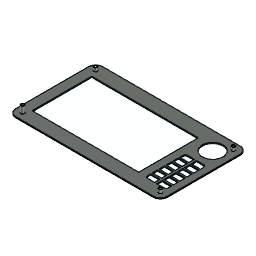
Nexus desk front (Autodesk Fusion 360 design; units mm, degrees)
part number: 2026-05-24-07-28-20-931
Autodesk Fusion 360 part; units mm, degrees
sketch "Sketch1" plane through (0, 0, 0) normal (0, 0, 1) x (1, 0, 0)
  line L0 (20, 40) -> (220, 40)
  line L1 (230, 30) -> (230, -76)
  line L2 (220, -86) -> (20, -86)
  line L3 (10, -76) -> (10, 30)
  arc A0 (20, 40) -> (10, 30) centre (20, 30) ccw
  arc A1 (230, 30) -> (220, 40) centre (220, 30) ccw
  arc A2 (10, -76) -> (20, -86) centre (20, -76) ccw
  arc A3 (220, -86) -> (230, -76) centre (220, -76) ccw
  line L4 (24.5203, 19.9433) -> (179.0203, 19.9433)
  line L5 (179.0203, 19.9433) -> (179.0203, -66.4567)
  line L6 (24.5203, 19.9433) -> (24.5203, -66.4567)
  line L7 (24.5203, -66.4567) -> (179.0203, -66.4567)
  circle A4 centre (205.8832, 13.8979) radius 15
  arc A5 (193, -10) -> (190, -13) centre (193, -13) ccw
  arc A6 (220, -13) -> (217, -10) centre (217, -13) ccw
  arc A7 (190, -64.7013) -> (193, -67.7013) centre (193, -64.7013) ccw
  arc A8 (217, -67.7013) -> (220, -64.7013) centre (217, -64.7013) ccw
  line L8 (203.1137, -60) -> (203.1137, -67.7013)
  line L9 (206.5757, -60) -> (206.5757, -67.7013)
  line L10 (190, -47.6988) -> (203.1137, -47.6988)
  line L11 (206.5757, -47.6988) -> (220, -47.6988)
  line L12 (190, -50) -> (203.1137, -50)
  line L13 (206.5757, -50) -> (220, -50)
  line L14 (203.1137, -50) -> (203.1137, -57.3154)
  line L15 (206.5757, -50) -> (206.5757, -57.3154)
  line L16 (190, -57.3154) -> (203.1137, -57.3154)
  line L17 (206.5757, -57.3154) -> (220, -57.3154)
  line L18 (190, -60) -> (203.1137, -60)
  line L19 (206.5757, -60) -> (220, -60)
  line L20 (190, -64.7013) -> (190, -60)
  line L21 (190, -57.3154) -> (190, -50)
  line L22 (190, -47.6988) -> (190, -40)
  line L23 (203.1137, -40) -> (203.1137, -47.6988)
  line L24 (190, -37.5051) -> (203.1137, -37.5051)
  line L25 (206.5757, -37.5051) -> (220, -37.5051)
  line L26 (190, -40) -> (203.1137, -40)
  line L27 (206.5757, -40) -> (220, -40)
  line L28 (206.5757, -40) -> (206.5757, -47.6988)
  line L29 (220, -50) -> (220, -57.3154)
  line L30 (220, -60) -> (220, -64.7013)
  line L31 (220, -40) -> (220, -47.6988)
  line L32 (193, -67.7013) -> (203.1137, -67.7013)
  line L33 (206.5757, -67.7013) -> (217, -67.7013)
  line L34 (203.1137, -30) -> (203.1137, -37.5051)
  line L35 (190, -27.6962) -> (203.1137, -27.6962)
  line L36 (206.5757, -27.6962) -> (220, -27.6962)
  line L37 (190, -30) -> (203.1137, -30)
  line L38 (206.5757, -30) -> (220, -30)
  line L39 (206.5757, -30) -> (206.5757, -37.5051)
  line L40 (220, -30) -> (220, -37.5051)
  line L41 (190, -37.5051) -> (190, -30)
  line L42 (190, -27.6962) -> (190, -20)
  line L43 (190, -17.8872) -> (190, -13)
  line L44 (203.1137, -10) -> (203.1137, -17.8872)
  line L45 (203.1137, -20) -> (203.1137, -27.6962)
  line L46 (190, -17.8872) -> (203.1137, -17.8872)
  line L47 (206.5757, -17.8872) -> (220, -17.8872)
  line L48 (190, -20) -> (203.1137, -20)
  line L49 (206.5757, -20) -> (220, -20)
  line L50 (206.5757, -10) -> (206.5757, -17.8872)
  line L51 (206.5757, -20) -> (206.5757, -27.6962)
  line L52 (220, -13) -> (220, -17.8872)
  line L53 (220, -20) -> (220, -27.6962)
  line L54 (193, -10) -> (203.1137, -10)
  line L55 (206.5757, -10) -> (217, -10)
  point P0 (10, 40)
  point P1 (230, 40)
  point P2 (10, -86)
  dimension "d1" = 220
  dimension "d2" = 126
  dimension "d3" = 10
  dimension "d4" = 10
  dimension "d5" = 10
  dimension "d6" = 154.5
  dimension "d7" = 86.4
  dimension "d8" = 86.4
  dimension "d9" = 30
  dimension "d10" = 3
  constraint horizontal L0
  constraint vertical L1
  constraint horizontal L2
  constraint vertical L3
  constraint coincident P0 L0
  constraint coincident P0 L3
  constraint tangent L0 A0
  constraint tangent L3 A0
  constraint coincident P1 L0
  constraint coincident P1 L1
  constraint tangent L0 A1
  constraint tangent L1 A1
  constraint coincident P2 L2
  constraint coincident P2 L3
  constraint tangent L2 A2
  constraint tangent L3 A2
  constraint tangent L1 A3
  constraint tangent L2 A3
  constraint equal A2 A3
  constraint perpendicular L3 L4
  constraint perpendicular L4 L5
  constraint perpendicular L4 L6
  constraint horizontal L54
  constraint vertical L52
  constraint vertical L20
  constraint perpendicular L47 L52
  constraint perpendicular L49 L53
  constraint perpendicular L36 L53
  constraint perpendicular L38 L40
  constraint perpendicular L25 L40
  constraint perpendicular L11 L31
  constraint perpendicular L13 L29
  constraint perpendicular L17 L29
  constraint perpendicular L19 L30
  constraint perpendicular L30 L33
  constraint perpendicular L8 L32
  constraint perpendicular L9 L19
  constraint tangent A5 L54
  constraint tangent A5 L43
  constraint tangent A6 L55
  constraint tangent A6 L52
  constraint equal A5 A6
  constraint tangent A7 L20
  constraint tangent A7 L32
  constraint equal A5 A7
  constraint tangent A8 L33
  constraint tangent A8 L30
  constraint equal A5 A8
  constraint collinear L8 L14
  constraint collinear L9 L15
  constraint collinear L10 L11
  constraint collinear L12 L13
  constraint collinear L14 L23
  constraint collinear L15 L28
  constraint collinear L16 L17
  constraint collinear L18 L19
  constraint collinear L20 L21
  constraint collinear L21 L22
  constraint collinear L22 L41
  constraint collinear L23 L34
  constraint collinear L24 L25
  constraint collinear L26 L27
  constraint collinear L28 L39
  constraint collinear L29 L31
  constraint collinear L29 L30
  constraint collinear L31 L40
  constraint collinear L32 L33
  constraint collinear L34 L45
  constraint collinear L35 L36
  constraint collinear L37 L38
  constraint collinear L39 L51
  constraint collinear L40 L53
  constraint collinear L41 L42
  constraint collinear L42 L43
  constraint collinear L44 L45
  constraint collinear L46 L47
  constraint collinear L48 L49
  constraint collinear L50 L51
  constraint collinear L52 L53
  constraint collinear L54 L55
  measures "d1" distance of P0 P1
  measures "d2" distance of P0 P2
  measures "d3" radius of A0
  measures "d4" radius of A1
  measures "d5" radius of A2
  measures "d6" distance of L4.start L4.end
  measures "d7" distance of L4.end L5.end
  measures "d8" distance of L4.start L6.end
  measures "d9" diameter of A4
  measures "d10" radius of A5
extrude "Extrude1" add sketch "Sketch1" along normal blind 1.5
sketch "Sketch2" plane through (0, 0, 1.5) normal (0, 0, 1) x (-1, 0, 0)
  arc A0 (-190, 64.7013) -> (-193, 67.7013) centre (-193, 64.7013) ccw
  line L0 (-190, 64.7013) -> (-190, 60)
  line L1 (-190, 60) -> (-203.1137, 60)
  line L2 (-203.1137, 60) -> (-203.1137, 67.7013)
  line L3 (-203.1137, 67.7013) -> (-193, 67.7013)
  line L4 (-206.5757, 57.3154) -> (-206.5757, 50)
  line L5 (-206.5757, 50) -> (-220, 50)
  line L6 (-220, 50) -> (-220, 57.3154)
  line L7 (-220, 57.3154) -> (-206.5757, 57.3154)
  line L8 (-203.1137, 57.3154) -> (-190, 57.3154)
  line L9 (-190, 57.3154) -> (-190, 50)
  line L10 (-190, 50) -> (-203.1137, 50)
  line L11 (-203.1137, 50) -> (-203.1137, 57.3154)
  arc A1 (-10, 76) -> (-20, 86) centre (-20, 76) ccw
  line L12 (-20, 86) -> (-220, 86)
  arc A2 (-220, 86) -> (-230, 76) centre (-220, 76) ccw
  line L13 (-230, 76) -> (-230, -30)
  arc A3 (-230, -30) -> (-220, -40) centre (-220, -30) ccw
  line L14 (-220, -40) -> (-20, -40)
  arc A4 (-20, -40) -> (-10, -30) centre (-20, -30) ccw
  line L15 (-10, -30) -> (-10, 76)
  line L16 (-24.5203, 66.4567) -> (-24.5203, -19.9433)
  line L17 (-24.5203, -19.9433) -> (-179.0203, -19.9433)
  line L18 (-179.0203, -19.9433) -> (-179.0203, 66.4567)
  line L19 (-179.0203, 66.4567) -> (-24.5203, 66.4567)
  circle A5 centre (-205.8832, -13.8979) radius 15
  line L20 (-220, 17.8872) -> (-206.5757, 17.8872)
  line L21 (-206.5757, 17.8872) -> (-206.5757, 10)
  line L22 (-206.5757, 10) -> (-217, 10)
  arc A6 (-220, 13) -> (-217, 10) centre (-217, 13) ccw
  line L23 (-220, 13) -> (-220, 17.8872)
  line L24 (-203.1137, 17.8872) -> (-190, 17.8872)
  line L25 (-190, 17.8872) -> (-190, 13)
  arc A7 (-193, 10) -> (-190, 13) centre (-193, 13) ccw
  line L26 (-193, 10) -> (-203.1137, 10)
  line L27 (-203.1137, 10) -> (-203.1137, 17.8872)
  line L28 (-206.5757, 27.6962) -> (-206.5757, 20)
  line L29 (-206.5757, 20) -> (-220, 20)
  line L30 (-220, 20) -> (-220, 27.6962)
  line L31 (-220, 27.6962) -> (-206.5757, 27.6962)
  line L32 (-203.1137, 27.6962) -> (-190, 27.6962)
  line L33 (-190, 27.6962) -> (-190, 20)
  line L34 (-190, 20) -> (-203.1137, 20)
  line L35 (-203.1137, 20) -> (-203.1137, 27.6962)
  line L36 (-206.5757, 37.5051) -> (-206.5757, 30)
  line L37 (-206.5757, 30) -> (-220, 30)
  line L38 (-220, 30) -> (-220, 37.5051)
  line L39 (-220, 37.5051) -> (-206.5757, 37.5051)
  line L40 (-206.5757, 67.7013) -> (-206.5757, 60)
  line L41 (-206.5757, 60) -> (-220, 60)
  line L42 (-220, 60) -> (-220, 64.7013)
  arc A8 (-217, 67.7013) -> (-220, 64.7013) centre (-217, 64.7013) ccw
  line L43 (-217, 67.7013) -> (-206.5757, 67.7013)
  line L44 (-206.5757, 47.6988) -> (-206.5757, 40)
  line L45 (-206.5757, 40) -> (-220, 40)
  line L46 (-220, 40) -> (-220, 47.6988)
  line L47 (-220, 47.6988) -> (-206.5757, 47.6988)
  line L48 (-203.1137, 37.5051) -> (-190, 37.5051)
  line L49 (-190, 37.5051) -> (-190, 30)
  line L50 (-190, 30) -> (-203.1137, 30)
  line L51 (-203.1137, 30) -> (-203.1137, 37.5051)
  line L52 (-203.1137, 47.6988) -> (-190, 47.6988)
  line L53 (-190, 47.6988) -> (-190, 40)
  line L54 (-190, 40) -> (-203.1137, 40)
  line L55 (-203.1137, 40) -> (-203.1137, 47.6988)
  circle A9 centre (-20, -30) radius 2.5
  circle A10 centre (-220, -30) radius 2.5
  circle A11 centre (-20, 80) radius 2.5
  circle A12 centre (-220, 80) radius 2.5
  dimension "d13" = 5
  dimension "d14" = 5
  dimension "d15" = 5
  dimension "d16" = 5
  constraint concentric A4 A9
  constraint concentric A3 A10
  measures "d13" diameter of A9
  measures "d14" diameter of A10
  measures "d15" diameter of A11
  measures "d16" diameter of A12
extrude "Extrude2" add sketch "Sketch2" along normal blind 5 contours A9
sketch "Sketch3" plane through (0, 0, 1.5) normal (0, 0, 1) x (-1, 0, 0)
  line L0 (-203.1137, 47.6988) -> (-190, 47.6988)
  line L1 (-190, 47.6988) -> (-190, 40)
  line L2 (-190, 40) -> (-203.1137, 40)
  line L3 (-203.1137, 40) -> (-203.1137, 47.6988)
  line L4 (-203.1137, 37.5051) -> (-190, 37.5051)
  line L5 (-190, 37.5051) -> (-190, 30)
  line L6 (-190, 30) -> (-203.1137, 30)
  line L7 (-203.1137, 30) -> (-203.1137, 37.5051)
  line L8 (-206.5757, 47.6988) -> (-206.5757, 40)
  line L9 (-206.5757, 40) -> (-220, 40)
  line L10 (-220, 40) -> (-220, 47.6988)
  line L11 (-220, 47.6988) -> (-206.5757, 47.6988)
  line L12 (-206.5757, 67.7013) -> (-206.5757, 60)
  line L13 (-206.5757, 60) -> (-220, 60)
  line L14 (-220, 60) -> (-220, 64.7013)
  arc A0 (-217, 67.7013) -> (-220, 64.7013) centre (-217, 64.7013) ccw
  line L15 (-217, 67.7013) -> (-206.5757, 67.7013)
  line L16 (-206.5757, 37.5051) -> (-206.5757, 30)
  line L17 (-206.5757, 30) -> (-220, 30)
  line L18 (-220, 30) -> (-220, 37.5051)
  line L19 (-220, 37.5051) -> (-206.5757, 37.5051)
  line L20 (-203.1137, 27.6962) -> (-190, 27.6962)
  line L21 (-190, 27.6962) -> (-190, 20)
  line L22 (-190, 20) -> (-203.1137, 20)
  line L23 (-203.1137, 20) -> (-203.1137, 27.6962)
  line L24 (-206.5757, 27.6962) -> (-206.5757, 20)
  line L25 (-206.5757, 20) -> (-220, 20)
  line L26 (-220, 20) -> (-220, 27.6962)
  line L27 (-220, 27.6962) -> (-206.5757, 27.6962)
  line L28 (-203.1137, 17.8872) -> (-190, 17.8872)
  line L29 (-190, 17.8872) -> (-190, 13)
  arc A1 (-193, 10) -> (-190, 13) centre (-193, 13) ccw
  line L30 (-193, 10) -> (-203.1137, 10)
  line L31 (-203.1137, 10) -> (-203.1137, 17.8872)
  line L32 (-220, 17.8872) -> (-206.5757, 17.8872)
  line L33 (-206.5757, 17.8872) -> (-206.5757, 10)
  line L34 (-206.5757, 10) -> (-217, 10)
  arc A2 (-220, 13) -> (-217, 10) centre (-217, 13) ccw
  line L35 (-220, 13) -> (-220, 17.8872)
  circle A3 centre (-205.8832, -13.8979) radius 15
  line L36 (-24.5203, 66.4567) -> (-24.5203, -19.9433)
  line L37 (-24.5203, -19.9433) -> (-179.0203, -19.9433)
  line L38 (-179.0203, -19.9433) -> (-179.0203, 66.4567)
  line L39 (-179.0203, 66.4567) -> (-24.5203, 66.4567)
  arc A4 (-10, 76) -> (-20, 86) centre (-20, 76) ccw
  line L40 (-20, 86) -> (-220, 86)
  arc A5 (-220, 86) -> (-230, 76) centre (-220, 76) ccw
  line L41 (-230, 76) -> (-230, -30)
  arc A6 (-230, -30) -> (-220, -40) centre (-220, -30) ccw
  line L42 (-220, -40) -> (-20, -40)
  arc A7 (-20, -40) -> (-10, -30) centre (-20, -30) ccw
  line L43 (-10, -30) -> (-10, 76)
  line L44 (-203.1137, 57.3154) -> (-190, 57.3154)
  line L45 (-190, 57.3154) -> (-190, 50)
  line L46 (-190, 50) -> (-203.1137, 50)
  line L47 (-203.1137, 50) -> (-203.1137, 57.3154)
  line L48 (-206.5757, 57.3154) -> (-206.5757, 50)
  line L49 (-206.5757, 50) -> (-220, 50)
  line L50 (-220, 50) -> (-220, 57.3154)
  line L51 (-220, 57.3154) -> (-206.5757, 57.3154)
  arc A8 (-190, 64.7013) -> (-193, 67.7013) centre (-193, 64.7013) ccw
  line L52 (-190, 64.7013) -> (-190, 60)
  line L53 (-190, 60) -> (-203.1137, 60)
  line L54 (-203.1137, 60) -> (-203.1137, 67.7013)
  line L55 (-203.1137, 67.7013) -> (-193, 67.7013)
  circle A9 centre (-20, -30) radius 2.5
  circle A10 centre (-220, -30) radius 2.5
  dimension "d19" = 5
  constraint concentric A6 A10
  measures "d19" diameter of A10
extrude "Extrude3" add sketch "Sketch3" along normal blind 5 contours A10
sketch "Sketch4" plane through (0, 0, 1.5) normal (0, 0, 1) x (-1, 0, 0)
  circle A0 centre (-20, -30) radius 2.5
  arc A1 (-190, 64.7013) -> (-193, 67.7013) centre (-193, 64.7013) ccw
  line L0 (-190, 64.7013) -> (-190, 60)
  line L1 (-190, 60) -> (-203.1137, 60)
  line L2 (-203.1137, 60) -> (-203.1137, 67.7013)
  line L3 (-203.1137, 67.7013) -> (-193, 67.7013)
  line L4 (-206.5757, 57.3154) -> (-206.5757, 50)
  line L5 (-206.5757, 50) -> (-220, 50)
  line L6 (-220, 50) -> (-220, 57.3154)
  line L7 (-220, 57.3154) -> (-206.5757, 57.3154)
  line L8 (-203.1137, 57.3154) -> (-190, 57.3154)
  line L9 (-190, 57.3154) -> (-190, 50)
  line L10 (-190, 50) -> (-203.1137, 50)
  line L11 (-203.1137, 50) -> (-203.1137, 57.3154)
  arc A2 (-10, 76) -> (-20, 86) centre (-20, 76) ccw
  line L12 (-20, 86) -> (-220, 86)
  arc A3 (-220, 86) -> (-230, 76) centre (-220, 76) ccw
  line L13 (-230, 76) -> (-230, -30)
  arc A4 (-230, -30) -> (-220, -40) centre (-220, -30) ccw
  line L14 (-220, -40) -> (-20, -40)
  arc A5 (-20, -40) -> (-10, -30) centre (-20, -30) ccw
  line L15 (-10, -30) -> (-10, 76)
  line L16 (-24.5203, 66.4567) -> (-24.5203, -19.9433)
  line L17 (-24.5203, -19.9433) -> (-179.0203, -19.9433)
  line L18 (-179.0203, -19.9433) -> (-179.0203, 66.4567)
  line L19 (-179.0203, 66.4567) -> (-24.5203, 66.4567)
  circle A6 centre (-205.8832, -13.8979) radius 15
  line L20 (-220, 17.8872) -> (-206.5757, 17.8872)
  line L21 (-206.5757, 17.8872) -> (-206.5757, 10)
  line L22 (-206.5757, 10) -> (-217, 10)
  arc A7 (-220, 13) -> (-217, 10) centre (-217, 13) ccw
  line L23 (-220, 13) -> (-220, 17.8872)
  line L24 (-203.1137, 17.8872) -> (-190, 17.8872)
  line L25 (-190, 17.8872) -> (-190, 13)
  arc A8 (-193, 10) -> (-190, 13) centre (-193, 13) ccw
  line L26 (-193, 10) -> (-203.1137, 10)
  line L27 (-203.1137, 10) -> (-203.1137, 17.8872)
  line L28 (-206.5757, 27.6962) -> (-206.5757, 20)
  line L29 (-206.5757, 20) -> (-220, 20)
  line L30 (-220, 20) -> (-220, 27.6962)
  line L31 (-220, 27.6962) -> (-206.5757, 27.6962)
  line L32 (-203.1137, 27.6962) -> (-190, 27.6962)
  line L33 (-190, 27.6962) -> (-190, 20)
  line L34 (-190, 20) -> (-203.1137, 20)
  line L35 (-203.1137, 20) -> (-203.1137, 27.6962)
  line L36 (-206.5757, 37.5051) -> (-206.5757, 30)
  line L37 (-206.5757, 30) -> (-220, 30)
  line L38 (-220, 30) -> (-220, 37.5051)
  line L39 (-220, 37.5051) -> (-206.5757, 37.5051)
  line L40 (-206.5757, 67.7013) -> (-206.5757, 60)
  line L41 (-206.5757, 60) -> (-220, 60)
  line L42 (-220, 60) -> (-220, 64.7013)
  arc A9 (-217, 67.7013) -> (-220, 64.7013) centre (-217, 64.7013) ccw
  line L43 (-217, 67.7013) -> (-206.5757, 67.7013)
  line L44 (-206.5757, 47.6988) -> (-206.5757, 40)
  line L45 (-206.5757, 40) -> (-220, 40)
  line L46 (-220, 40) -> (-220, 47.6988)
  line L47 (-220, 47.6988) -> (-206.5757, 47.6988)
  line L48 (-203.1137, 37.5051) -> (-190, 37.5051)
  line L49 (-190, 37.5051) -> (-190, 30)
  line L50 (-190, 30) -> (-203.1137, 30)
  line L51 (-203.1137, 30) -> (-203.1137, 37.5051)
  line L52 (-203.1137, 47.6988) -> (-190, 47.6988)
  line L53 (-190, 47.6988) -> (-190, 40)
  line L54 (-190, 40) -> (-203.1137, 40)
  line L55 (-203.1137, 40) -> (-203.1137, 47.6988)
  circle A10 centre (-220, -30) radius 2.5
  circle A11 centre (-20, 80) radius 2.5
  dimension "d22" = 5
  measures "d22" diameter of A11
extrude "Extrude4" add sketch "Sketch4" along normal blind 5 contours A11
sketch "Sketch5" plane through (0, 0, 1.5) normal (0, 0, 1) x (-1, 0, 0)
  circle A0 centre (-220, -30) radius 2.5
  line L0 (-203.1137, 47.6988) -> (-190, 47.6988)
  line L1 (-190, 47.6988) -> (-190, 40)
  line L2 (-190, 40) -> (-203.1137, 40)
  line L3 (-203.1137, 40) -> (-203.1137, 47.6988)
  line L4 (-203.1137, 37.5051) -> (-190, 37.5051)
  line L5 (-190, 37.5051) -> (-190, 30)
  line L6 (-190, 30) -> (-203.1137, 30)
  line L7 (-203.1137, 30) -> (-203.1137, 37.5051)
  line L8 (-206.5757, 47.6988) -> (-206.5757, 40)
  line L9 (-206.5757, 40) -> (-220, 40)
  line L10 (-220, 40) -> (-220, 47.6988)
  line L11 (-220, 47.6988) -> (-206.5757, 47.6988)
  line L12 (-206.5757, 67.7013) -> (-206.5757, 60)
  line L13 (-206.5757, 60) -> (-220, 60)
  line L14 (-220, 60) -> (-220, 64.7013)
  arc A1 (-217, 67.7013) -> (-220, 64.7013) centre (-217, 64.7013) ccw
  line L15 (-217, 67.7013) -> (-206.5757, 67.7013)
  line L16 (-206.5757, 37.5051) -> (-206.5757, 30)
  line L17 (-206.5757, 30) -> (-220, 30)
  line L18 (-220, 30) -> (-220, 37.5051)
  line L19 (-220, 37.5051) -> (-206.5757, 37.5051)
  line L20 (-203.1137, 27.6962) -> (-190, 27.6962)
  line L21 (-190, 27.6962) -> (-190, 20)
  line L22 (-190, 20) -> (-203.1137, 20)
  line L23 (-203.1137, 20) -> (-203.1137, 27.6962)
  line L24 (-206.5757, 27.6962) -> (-206.5757, 20)
  line L25 (-206.5757, 20) -> (-220, 20)
  line L26 (-220, 20) -> (-220, 27.6962)
  line L27 (-220, 27.6962) -> (-206.5757, 27.6962)
  line L28 (-203.1137, 17.8872) -> (-190, 17.8872)
  line L29 (-190, 17.8872) -> (-190, 13)
  arc A2 (-193, 10) -> (-190, 13) centre (-193, 13) ccw
  line L30 (-193, 10) -> (-203.1137, 10)
  line L31 (-203.1137, 10) -> (-203.1137, 17.8872)
  line L32 (-220, 17.8872) -> (-206.5757, 17.8872)
  line L33 (-206.5757, 17.8872) -> (-206.5757, 10)
  line L34 (-206.5757, 10) -> (-217, 10)
  arc A3 (-220, 13) -> (-217, 10) centre (-217, 13) ccw
  line L35 (-220, 13) -> (-220, 17.8872)
  circle A4 centre (-205.8832, -13.8979) radius 15
  line L36 (-24.5203, 66.4567) -> (-24.5203, -19.9433)
  line L37 (-24.5203, -19.9433) -> (-179.0203, -19.9433)
  line L38 (-179.0203, -19.9433) -> (-179.0203, 66.4567)
  line L39 (-179.0203, 66.4567) -> (-24.5203, 66.4567)
  arc A5 (-10, 76) -> (-20, 86) centre (-20, 76) ccw
  line L40 (-20, 86) -> (-220, 86)
  arc A6 (-220, 86) -> (-230, 76) centre (-220, 76) ccw
  line L41 (-230, 76) -> (-230, -30)
  arc A7 (-230, -30) -> (-220, -40) centre (-220, -30) ccw
  line L42 (-220, -40) -> (-20, -40)
  arc A8 (-20, -40) -> (-10, -30) centre (-20, -30) ccw
  line L43 (-10, -30) -> (-10, 76)
  line L44 (-203.1137, 57.3154) -> (-190, 57.3154)
  line L45 (-190, 57.3154) -> (-190, 50)
  line L46 (-190, 50) -> (-203.1137, 50)
  line L47 (-203.1137, 50) -> (-203.1137, 57.3154)
  line L48 (-206.5757, 57.3154) -> (-206.5757, 50)
  line L49 (-206.5757, 50) -> (-220, 50)
  line L50 (-220, 50) -> (-220, 57.3154)
  line L51 (-220, 57.3154) -> (-206.5757, 57.3154)
  arc A9 (-190, 64.7013) -> (-193, 67.7013) centre (-193, 64.7013) ccw
  line L52 (-190, 64.7013) -> (-190, 60)
  line L53 (-190, 60) -> (-203.1137, 60)
  line L54 (-203.1137, 60) -> (-203.1137, 67.7013)
  line L55 (-203.1137, 67.7013) -> (-193, 67.7013)
  circle A10 centre (-20, -30) radius 2.5
  circle A11 centre (-20, 80) radius 2.5
  circle A12 centre (-220, 80) radius 2.5
  dimension "d25" = 5
  measures "d25" diameter of A12
extrude "Extrude5" add sketch "Sketch5" along normal blind 5 contours A12
sketch "Sketch6" plane through (0, 0, 1.5) normal (0, 0, 1) x (-1, 0, 0)
  circle A0 centre (-20, -30) radius 2.5
  arc A1 (-190, 64.7013) -> (-193, 67.7013) centre (-193, 64.7013) ccw
  line L0 (-190, 64.7013) -> (-190, 60)
  line L1 (-190, 60) -> (-203.1137, 60)
  line L2 (-203.1137, 60) -> (-203.1137, 67.7013)
  line L3 (-203.1137, 67.7013) -> (-193, 67.7013)
  line L4 (-206.5757, 57.3154) -> (-206.5757, 50)
  line L5 (-206.5757, 50) -> (-220, 50)
  line L6 (-220, 50) -> (-220, 57.3154)
  line L7 (-220, 57.3154) -> (-206.5757, 57.3154)
  line L8 (-203.1137, 57.3154) -> (-190, 57.3154)
  line L9 (-190, 57.3154) -> (-190, 50)
  line L10 (-190, 50) -> (-203.1137, 50)
  line L11 (-203.1137, 50) -> (-203.1137, 57.3154)
  arc A2 (-10, 76) -> (-20, 86) centre (-20, 76) ccw
  line L12 (-20, 86) -> (-220, 86)
  arc A3 (-220, 86) -> (-230, 76) centre (-220, 76) ccw
  line L13 (-230, 76) -> (-230, -30)
  arc A4 (-230, -30) -> (-220, -40) centre (-220, -30) ccw
  line L14 (-220, -40) -> (-20, -40)
  arc A5 (-20, -40) -> (-10, -30) centre (-20, -30) ccw
  line L15 (-10, -30) -> (-10, 76)
  line L16 (-24.5203, 66.4567) -> (-24.5203, -19.9433)
  line L17 (-24.5203, -19.9433) -> (-179.0203, -19.9433)
  line L18 (-179.0203, -19.9433) -> (-179.0203, 66.4567)
  line L19 (-179.0203, 66.4567) -> (-24.5203, 66.4567)
  circle A6 centre (-205.8832, -13.8979) radius 15
  line L20 (-220, 17.8872) -> (-206.5757, 17.8872)
  line L21 (-206.5757, 17.8872) -> (-206.5757, 10)
  line L22 (-206.5757, 10) -> (-217, 10)
  arc A7 (-220, 13) -> (-217, 10) centre (-217, 13) ccw
  line L23 (-220, 13) -> (-220, 17.8872)
  line L24 (-203.1137, 17.8872) -> (-190, 17.8872)
  line L25 (-190, 17.8872) -> (-190, 13)
  arc A8 (-193, 10) -> (-190, 13) centre (-193, 13) ccw
  line L26 (-193, 10) -> (-203.1137, 10)
  line L27 (-203.1137, 10) -> (-203.1137, 17.8872)
  line L28 (-206.5757, 27.6962) -> (-206.5757, 20)
  line L29 (-206.5757, 20) -> (-220, 20)
  line L30 (-220, 20) -> (-220, 27.6962)
  line L31 (-220, 27.6962) -> (-206.5757, 27.6962)
  line L32 (-203.1137, 27.6962) -> (-190, 27.6962)
  line L33 (-190, 27.6962) -> (-190, 20)
  line L34 (-190, 20) -> (-203.1137, 20)
  line L35 (-203.1137, 20) -> (-203.1137, 27.6962)
  line L36 (-206.5757, 37.5051) -> (-206.5757, 30)
  line L37 (-206.5757, 30) -> (-220, 30)
  line L38 (-220, 30) -> (-220, 37.5051)
  line L39 (-220, 37.5051) -> (-206.5757, 37.5051)
  line L40 (-206.5757, 67.7013) -> (-206.5757, 60)
  line L41 (-206.5757, 60) -> (-220, 60)
  line L42 (-220, 60) -> (-220, 64.7013)
  arc A9 (-217, 67.7013) -> (-220, 64.7013) centre (-217, 64.7013) ccw
  line L43 (-217, 67.7013) -> (-206.5757, 67.7013)
  line L44 (-206.5757, 47.6988) -> (-206.5757, 40)
  line L45 (-206.5757, 40) -> (-220, 40)
  line L46 (-220, 40) -> (-220, 47.6988)
  line L47 (-220, 47.6988) -> (-206.5757, 47.6988)
  line L48 (-203.1137, 37.5051) -> (-190, 37.5051)
  line L49 (-190, 37.5051) -> (-190, 30)
  line L50 (-190, 30) -> (-203.1137, 30)
  line L51 (-203.1137, 30) -> (-203.1137, 37.5051)
  line L52 (-203.1137, 47.6988) -> (-190, 47.6988)
  line L53 (-190, 47.6988) -> (-190, 40)
  line L54 (-190, 40) -> (-203.1137, 40)
  line L55 (-203.1137, 40) -> (-203.1137, 47.6988)
  circle A10 centre (-220, -30) radius 2.5
sketch "Sketch7" plane through (0, 0, 1.5) normal (0, 0, 1) x (-1, 0, 0)
delete_face "DeleteFace1" 2 faces at (219.0183, -80.5668, 6.5) (219.3229, -82.4066, 4.8333)
delete_face "DeleteFace2" 2 faces at (18.0732, -80.3303, 6.5) (22.3492, -79.1449, 4.8333)
sketch "Sketch8" plane through (0, 0, 1.5) normal (0, 0, 1) x (-1, 0, 0)
  circle A0 centre (-220, 76) radius 2.5
  circle A1 centre (-20, 76) radius 2.5
  dimension "d28" = 5
  dimension "d29" = 5
  measures "d28" diameter of A0
  measures "d29" diameter of A1
extrude "Extrude6" add sketch "Sketch8" along normal blind 5 contours A0
sketch "Sketch9" plane through (0, 0, 1.5) normal (0, 0, 1) x (-1, 0, 0)
sketch "Sketch10" plane through (0, 0, 1.5) normal (0, 0, 1) x (-1, 0, 0)
  circle A0 centre (-20, 76) radius 2.5
  dimension "d32" = 5
  measures "d32" diameter of A0
extrude "Extrude7" add sketch "Sketch10" along normal blind 10
sketch "Sketch11" plane through (0, 0, 1.5) normal (0, 0, 1) x (-1, 0, 0)
form "Form1" [no effect]
sketch "Sketch12" plane through (0, 0, 6.5) normal (0, 0, 1) x (-1, 0, 0)
  circle A0 centre (-220, 76) radius 2.5
  circle A1 through (-18, -30, -5) (-21, -28.2679, -5) (-21, -31.7321, -5)
  circle A2 through (-218, -30, -5) (-221, -28.2679, -5) (-221, -31.7321, -5)
  circle A3 centre (-220, 76) radius 2
  circle A4 through (-18, 76, -5) (-21, 77.732, -5) (-21, 74.2679, -5)
  dimension "d35" = 4
  dimension "d36" = 4
  dimension "d37" = 4
  dimension "d38" = 4
  constraint concentric A0 A3
  measures "d37" diameter of A3
sketch "Sketch13" plane through (0, 0, 6.5) normal (0, 0, 1) x (-1, 0, 0)
  circle A0 centre (-20, -30) radius 2.5
  circle A1 centre (-20, -30) radius 2
  circle A2 centre (-220, -30) radius 2
  circle A3 centre (-20, 76) radius 2
  dimension "d39" = 4
  dimension "d40" = 4
  dimension "d41" = 4
  constraint concentric A0 A1
  measures "d39" diameter of A1
  measures "d40" diameter of A2
  measures "d41" diameter of A3
extrude "Extrude8" cut sketch "Sketch13" sketch "Sketch12" against normal blind 30 contours A1 | A2 of sketch 2 contours A3
sketch "Sketch14" plane through (0, 0, 11.5) normal (0, 0, 1) x (-1, 0, 0)
  circle A0 centre (-20, 76) radius 2.5
  circle A1 centre (-20, 76) radius 2
  dimension "d44" = 4
  constraint concentric A0 A1
  measures "d44" diameter of A1
extrude "Extrude9" cut sketch "Sketch14" against normal blind 40 contours A1
thread "Thread1" "ISO Metric profile 4.0 M4x0.7 M4x0.7 6H" major diameter 4.1095 minor diameter 3.332 pitch 0.7 angle 60 resizes the face on face at (21.843, -75.2231, 3.8333)
thread "Thread2" "ISO Metric profile 4.0 M4x0.7 M4x0.7 6H" major diameter 4.1095 minor diameter 3.332 pitch 0.7 angle 60 resizes the face on face at (18.0099, 30.1991, 2.1667)
thread "Thread3" "ISO Metric profile 4.0 M4x0.7 M4x0.7 6H" major diameter 4.1095 minor diameter 3.332 pitch 0.7 angle 60 resizes the face on face at (218.9149, 31.6801, 4.3333)
thread "Thread4" "ISO Metric profile 4.0 M4x0.7 M4x0.7 6H" major diameter 4.1095 minor diameter 3.332 pitch 0.7 angle 60 resizes the face on face at (218.6035, -77.4317, 4.3333)
